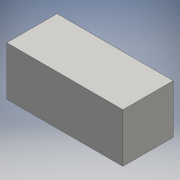
# Autodesk Inventor part: caja
Saved by Autodesk Inventor 2016 (Build 200138000, 138)
## iProperties
Created: 2017-12-31
Part Number: caja
Material: Genérico
Document SubType Name: Sheet Metal
Designer: David
Density: 1 g/cm^3
Sheet Metal Rule: Por defecto_mm
Appearance: Valor por defecto
Author: David
Autodesk Inventor part; units mm, degrees
ref_plane "YZ Plane" through (0, 0, 0) normal (1, 0, 0) x (0, 1, 0)
ref_plane "XZ Plane" through (0, 0, 0) normal (0, 1, 0) x (-1, 0, 0)
ref_plane "XY Plane" through (0, 0, 0) normal (0, 0, 1) x (1, 0, 0)
sketch "Boceto1" plane through (0, 0, 0) normal (0, 1, 0) x (-1, 0, 0)
  line L0 (0, 0) -> (-45, 0)
  line L1 (-45, 0) -> (-45, -19)
  line L2 (-45, -19) -> (0, -19)
  line L3 (0, -19) -> (0, 0)
  constraints: 8 end point, 2 parallel, 1 horizontal, 1 perpendicular
extrude "Extrusión1" add sketch "Boceto1" along normal blind 19.5
sketch "Boceto2" plane through (0, 19.5, 0) normal (0, 1, 0) x (1, 0, 0)
  line L0 (0, 19) -> (0, 0) projected
  line L1 (45, 0) -> (45, 19) projected
  line L2 (0, 0) -> (45, 0) projected
  line L3 (45, 19) -> (0, 19) projected
  line L4 (0.3, 0.3) -> (0.3, 9.5)
  line L5 (0.3, 0.3) -> (12.3526, 0.3)
  line L6 (0.3, 9.5) -> (0.3, 18.7)
  line L7 (0.3, 18.7) -> (13.3767, 18.7)
  line L8 (13.3767, 18.7) -> (25.3714, 18.7)
  line L9 (25.3714, 18.7) -> (38.8857, 18.7)
  line L10 (44.7, 0.3) -> (44.7, 18.7)
  line L11 (44.7, 18.7) -> (38.8857, 18.7)
  line L12 (44.7, 0.3) -> (33.7568, 0.3)
  line L13 (12.3526, 0.3) -> (33.7568, 0.3)
  constraints: 20 end point, 4 parallel, 3 horizontal, 2 vertical, 1 collinear
extrude "Extrusión2" cut sketch "Boceto2" against normal blind 19 contours L4 L6 L7 L8 L9 L11 L10 L12 L13 L5
equation "\"Radio_pliegue\" = Grosor"
equation "\"Anchura_desahogo_plegado\" = Grosor"
equation "\"Profundidad_desahogo_plegado\" = 0.5 * Grosor"
equation "\"Tamaño_destalonado\" = 4 * Grosor"
equation "\"Remanente_mínimo\" = 2 * Grosor"
equation "\"Radiodetransición\" = Radio_pliegue"
equation "\"Tamaño_de_radio_de_Jacobi\" = Radio_pliegue"
equation "\"TamañoSeparación\" = Grosor"
equation "\"Grosor\" = 0.5"
